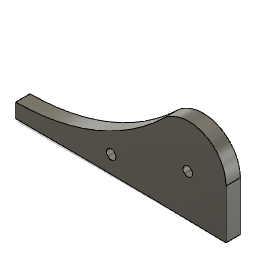
End_Block_Original_1_Public_v4 (Autodesk Fusion 360 design; units mm, degrees)
Autodesk Fusion 360 part; units mm, degrees
sketch "End Block Outline" plane through (0, 0, 0) normal (0, 0, 1) x (1, 0, 0)
  line L0 (0, 0) -> (0, 19.05)
  line L1 (0, 0) -> (279.4, 0) construction
  arc A0 (279.4, -3.123) -> (0, 0) centre (0, -12500) ccw
  arc A1 (0, 19.05) -> (195.4998, 97.9237) centre (0, 300.7741) ccw
  line L2 (0, 19.05) -> (279.4, 19.05) construction
  line L3 (279.4, 0) -> (279.4, -3.123) construction
  arc A2 (279.4, 62.2608) -> (195.4998, 97.9237) centre (229.8704, 62.2608) ccw
  line L4 (279.4, 62.2608) -> (279.4, -3.123)
  circle A3 centre (127, 22.225) radius 6.35
  circle A4 centre (228.6, 53.7591) radius 6.35
  line L5 (170, 19.05) -> (170, 76.1222) construction
  dimension "EndThickness" = 19.05
  dimension "BaseRadius" = 12500
  dimension "ArcRadius" = 281.7241
  dimension "BlockWidth" = 279.4
  dimension "ArcCordLength" = 210.8109
  dimension "d13" = 12.7
  dimension "d14" = 127
  dimension "d15" = 22.225
  dimension "d16" = 101.6
  dimension "d17" = 31.5341
  dimension "TestLength" = 170
  dimension "d2" = 65.002
  constraint coincident L0.start L1.start
  constraint perpendicular L0 L1
  constraint horizontal L1
  constraint tangent L1 A0
  constraint perpendicular L0 L2
  constraint tangent A1 L2
  constraint perpendicular L1 L3
  constraint coincident A0 L3.end
  constraint tangent A1 A2
  constraint perpendicular L1 L4
  constraint tangent A2 L4
  constraint equal A3 A4
  constraint coincident L2.end L4
  constraint coincident L2 L5.start
  constraint coincident A1 L5.end
  constraint perpendicular L2 L5
  measures "EndThickness" distance of L0.start L0.end
  measures "BaseRadius" radius of A0
  measures "ArcRadius" radius of A1
  measures "BlockWidth" horizontal distance of L0.start L1.end
  measures "ArcCordLength" distance of L0.end A1.end
  measures "d13" diameter of A3
  measures "d14" horizontal distance of L0.end A3.centre
  measures "d15" distance of L1 A3.centre
  measures "d16" horizontal distance of A3.centre A4.centre
  measures "d17" vertical distance of A3.centre A4.centre
  measures "TestLength" distance of L0.end L5.start
extrude "Extrude1" add sketch "End Block Outline" along normal blind 19.05
equation "BlockWidth = 11\""
equation "ArcCordLength = 2 * ArcRadius * sin(ArcAngle / 2)"
equation "d14 = 5\""
equation "d15 = ( 7 / 8 ) * 1\""
equation "d16 = 4\""
equation "ArcLength = 216.06764 mm"
equation "ArcAngle = ( 360 * ArcLength / ( 2 * PI * ArcRadius ) ) * 1 deg" comment "Internal computation"
named bodies: "End Block"
